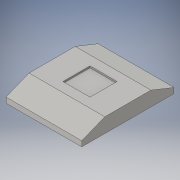
# Autodesk Inventor part: monitor (for assembly)
Saved by Autodesk Inventor 2016 (Build 200138000, 138)
## iProperties
Created: 2017-10-23
Part Number: monitor (for assembly)
Material: Generic
Document SubType Name: Modeling
Designer: student
Density: 1 g/cm^3
Appearance: Default
Author: student
Autodesk Inventor part; units mm, degrees
ref_plane "YZ Plane" through (0, 0, 0) normal (1, 0, 0) x (0, 1, 0)
ref_plane "XZ Plane" through (0, 0, 0) normal (0, 1, 0) x (-1, 0, 0)
ref_plane "XY Plane" through (0, 0, 0) normal (0, 0, 1) x (1, 0, 0)
sketch "Sketch1" plane through (0, 0, 0) normal (0, 1, 0) x (-1, 0, 0)
  line L0 (-168.91, 205.74) -> (168.91, 205.74)
  line L1 (168.91, 205.74) -> (168.91, -205.74)
  line L2 (168.91, -205.74) -> (-168.91, -205.74)
  line L3 (-168.91, -205.74) -> (-168.91, 205.74)
  line L4 (-168.91, 205.74) -> (168.91, -205.74) construction
  line L5 (168.91, 205.74) -> (-168.91, -205.74) construction
  point P0 (0, 0)
  dimension "d0" = 411.48
  dimension "d1" = 337.82
  constraints: 12 end point, 2 midpoint, 2 parallel, 1 horizontal, 1 perpendicular
  measures "d0" distance of L0.end L1.end
  measures "d1" distance of L1.end L2.end
extrude "Extrusion1" add sketch "Sketch1" along normal blind 65.024
sketch "Sketch2" plane through (168.91, 0, 205.74) normal (1, 0, 0) x (0, 0, -1)
  line L0 (102.87, 65.024) -> (308.61, 65.024)
  line L1 (411.48, 0) -> (411.48, 23.876)
  line L2 (308.61, 65.024) -> (411.48, 23.876)
  line L3 (411.48, 0) -> (411.48, 65.024) projected
  line L4 (308.61, 65.024) -> (411.48, 65.024)
  line L5 (411.48, 65.024) -> (411.48, 23.876)
  line L6 (102.87, 65.024) -> (0, 23.876)
  line L7 (0, 23.876) -> (0, 65.024)
  line L8 (0, 65.024) -> (102.87, 65.024)
  line L9 (411.48, 0) -> (0, 0) projected
  point P0 (205.74, 0)
  point P1 (205.74, 65.024)
  point P2 (205.74, 65.024)
  dimension "d4" = 205.74
  dimension "d5" = 23.876
  dimension "d6" = 23.876
  constraints: 16 end point, 2 perpendicular, 1 coincident, 1 horizontal, 1 midpoint
  measures "d4" distance of L0.start L0.end
  measures "d5" distance of L1.start L1.end
  measures "d6" distance from line of L9 L6.end
extrude "Extrusion2" cut sketch "Sketch2" against normal blind 387.2865
sketch "Sketch3" plane through (0, 65.024, 0) normal (0, 1, 0) x (1, 0, 0)
  line L0 (60.325, -60.325) -> (-60.325, -60.325)
  line L1 (-60.325, -60.325) -> (-60.325, 60.325)
  line L2 (-60.325, 60.325) -> (60.325, 60.325)
  line L3 (60.325, 60.325) -> (60.325, -60.325)
  line L4 (60.325, -60.325) -> (-60.325, 60.325) construction
  line L5 (-60.325, -60.325) -> (60.325, 60.325) construction
  point P0 (0, 0)
  dimension "d9" = 120.65
  dimension "d10" = 120.65
  constraints: 12 end point, 2 midpoint, 2 parallel, 1 horizontal, 1 perpendicular
  measures "d9" distance of L0.end L1.end
  measures "d10" distance of L1.end L2.end
extrude "Extrusion3" cut sketch "Sketch3" against normal blind 7.1437
body "Solid1"
